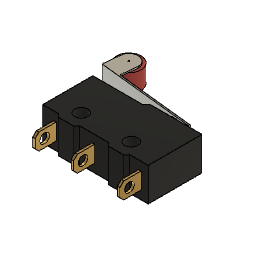
NO-NC Bump Switch (Autodesk Fusion 360 design; units mm, degrees)
Autodesk Fusion 360 part; units mm, degrees
sketch "Body" plane through (0, 0, 0) normal (0, 0, 1) x (1, 0, 0)
  line L0 (10, -5.1) -> (-10, -5.1)
  line L1 (-10, -5.1) -> (-10, 5.1)
  line L2 (-10, 5.1) -> (10, 5.1)
  line L3 (10, 5.1) -> (10, -5.1)
  line L4 (10, -5.1) -> (-10, 5.1) construction
  line L5 (-10, -5.1) -> (10, 5.1) construction
  line L6 (8.4, 5.1) -> (8.4, -5.1) construction
  line L7 (-0.4, 5.1) -> (-0.4, -5.1) construction
  line L8 (-7.7, 5.1) -> (-7.7, -5.1) construction
  line L9 (-7.7, -5.1) -> (-7.7, -9.1) construction
  line L10 (-0.4, -5.1) -> (-0.4, -9.1) construction
  line L11 (8.4, -5.1) -> (8.4, -9.1) construction
  line L12 (-10, -5.1) -> (10, -5.1) construction
  line L13 (10, -5.1) -> (10, -5.71) construction
  line L14 (10, -5.71) -> (-10, -5.71) construction
  line L15 (-10, -5.71) -> (-10, -5.1) construction
  line L16 (10, -2.81) -> (-10, -2.81) construction
  line L17 (-10, -2.81) -> (4.5, -2.81) construction
  circle A0 centre (4.5, -2.81) radius 1.25
  line L18 (4.5, -2.81) -> (-5, -2.81) construction
  circle A1 centre (-5, -2.81) radius 1.25
  line L19 (-5, -2.81) -> (-5, -5.71) construction
  line L20 (4.5, -2.81) -> (4.5, -5.71) construction
  line L21 (3, -5.71) -> (6, -5.71)
  line L22 (4.5, -5.1) -> (4.5, -5.71) construction
  line L23 (-5, -5.1) -> (-5, -5.71) construction
  line L24 (2.5, -5.1) -> (6.5, -5.1)
  line L25 (2.5, -5.1) -> (3, -5.71)
  line L26 (6, -5.71) -> (6.5, -5.1)
  line L27 (-6.5, -5.71) -> (-3.5, -5.71)
  line L28 (-7, -5.1) -> (-3, -5.1)
  line L29 (-7, -5.1) -> (-6.5, -5.71)
  line L30 (-3.5, -5.71) -> (-3, -5.1)
  line L31 (-7.465, -5.1) -> (-7.935, -5.1)
  line L32 (-7.935, -5.1) -> (-7.935, -9.1)
  line L33 (-7.935, -9.1) -> (-7.465, -9.1)
  line L34 (-7.465, -9.1) -> (-7.465, -5.1)
  line L35 (-7.465, -5.1) -> (-7.935, -9.1) construction
  line L36 (-7.935, -5.1) -> (-7.465, -9.1) construction
  line L37 (-0.165, -5.1) -> (-0.635, -5.1)
  line L38 (-0.635, -5.1) -> (-0.635, -9.1)
  line L39 (-0.635, -9.1) -> (-0.165, -9.1)
  line L40 (-0.165, -9.1) -> (-0.165, -5.1)
  line L41 (-0.165, -5.1) -> (-0.635, -9.1) construction
  line L42 (-0.635, -5.1) -> (-0.165, -9.1) construction
  line L43 (8.635, -5.1) -> (8.165, -5.1)
  line L44 (8.165, -5.1) -> (8.165, -9.1)
  line L45 (8.165, -9.1) -> (8.635, -9.1)
  line L46 (8.635, -9.1) -> (8.635, -5.1)
  line L47 (8.635, -5.1) -> (8.165, -9.1) construction
  line L48 (8.165, -5.1) -> (8.635, -9.1) construction
  line L49 (-10, -5.1) -> (-10, 4.38)
  line L50 (-10, 4.38) -> (-0.52, 4.38)
  line L51 (-0.52, 4.38) -> (0.0693, 5.1)
  line L52 (-0.52, 4.38) -> (0.4104, 4.38) construction
  point P0 (4.5, -5.1)
  point P1 (-7.7, -7.1)
  point P2 (-0.4, -7.1)
  point P3 (8.4, -7.1)
  dimension "d1" = 20
  dimension "d2" = 10.2
  dimension "d3" = 1.6
  dimension "d4" = 10.4
  dimension "d5" = 17.7
  dimension "d6" = 4
  dimension "d7" = 4
  dimension "d8" = 4
  dimension "d12" = 0.61
  dimension "d13" = 2.9
  dimension "d14" = 14.5
  dimension "d15" = 2.5
  dimension "d16" = 9.5
  dimension "d17" = 2.5
  dimension "d21" = 3
  dimension "d22" = 4
  dimension "d23" = 3
  dimension "d24" = 4
  dimension "d25" = 0.47
  dimension "d26" = 0.47
  dimension "d27" = 4
  dimension "d28" = 0.47
  dimension "d51" = 9.48
  dimension "d52" = 9.48
  dimension "d53" = 50.7
  constraint horizontal L0
  constraint perpendicular L0 L1
  constraint parallel L0 L2
  constraint parallel L1 L3
  constraint coincident L4 origin
  constraint coincident L5 origin
  constraint perpendicular L0 L9
  constraint perpendicular L0 L10
  constraint perpendicular L0 L11
  constraint horizontal L12
  constraint vertical L13
  constraint horizontal L14
  constraint vertical L15
  constraint coincident L0.start L3.end
  constraint perpendicular L8 L17
  constraint coincident L17.end A0.centre
  constraint parallel L16 L18
  constraint coincident L18.end A1.centre
  constraint coincident L14 L19.end
  constraint perpendicular L14 L19
  constraint coincident L14 L20.end
  constraint perpendicular L14 L20
  constraint coincident L20 P0
  constraint coincident L12 P0
  constraint horizontal L21
  constraint coincident P0 L22.start
  constraint coincident L19 L23.start
  constraint coincident L12 L23.start
  constraint horizontal L24
  constraint midpoint L20.end L21
  constraint midpoint P0 L24
  constraint horizontal L27
  constraint horizontal L28
  constraint midpoint L19.end L27
  constraint midpoint L23.start L28
  constraint horizontal L31
  constraint perpendicular L31 L32
  constraint parallel L31 L33
  constraint parallel L32 L34
  constraint coincident L35 P1
  constraint coincident L36 P1
  constraint midpoint L9 P1
  constraint horizontal L37
  constraint perpendicular L37 L38
  constraint parallel L37 L39
  constraint parallel L38 L40
  constraint coincident L41 P2
  constraint coincident L42 P2
  constraint midpoint L10 P2
  constraint horizontal L43
  constraint perpendicular L43 L44
  constraint parallel L43 L45
  constraint parallel L44 L46
  constraint coincident L47 P3
  constraint coincident L48 P3
  constraint midpoint L11 P3
  constraint perpendicular L16 L49
  constraint perpendicular L8 L50
  constraint horizontal L52
  constraint coincident L2 L51.end
  measures "d1" distance of L1.end L2.end
  measures "d2" distance of L0.end L1.end
  measures "d6" distance of L8.end L9.end
  measures "d7" distance of L7.end L10.end
  measures "d8" distance of L6.end L11.end
  measures "d12" distance of L0.end L14.end
  measures "d14" distance of L16.end L17.end
  measures "d15" diameter of A0
  measures "d16" distance of L17.end L18.end
  measures "d17" diameter of A1
  measures "d21" distance of L21.start L21.end
  measures "d22" distance of L24.start L24.end
  measures "d23" distance of L27.start L27.end
  measures "d24" distance of L28.start L28.end
  measures "d25" distance of L32.end L33.end
  measures "d26" distance of L38.end L39.end
  measures "d27" distance of L37.end L38.end
  measures "d28" distance of L44.end L45.end
  measures "d51" distance of L0.end L49.end
  measures "d52" distance of L49.end L50.end
  measures "d53" angle of L51 L52
sketch "Stem" plane through (0, 0, 0) normal (0, 0, 1) x (1, 0, 0)
  line L0 (2.8, 6.7) -> (3.4, 6.7)
  line L1 (4, 6.1) -> (4, 5.1)
  line L2 (4, 5.1) -> (2.2, 5.1)
  line L3 (2.2, 5.1) -> (2.2, 6.1)
  line L4 (10, 5.1) -> (10, -5.1) construction
  line L5 (10, 5.1) -> (3.1, 5.1) construction
  arc A0 (2.8, 6.7) -> (2.2, 6.1) centre (2.8, 6.1) ccw
  arc A1 (4, 6.1) -> (3.4, 6.7) centre (3.4, 6.1) ccw
  line L6 (10, 5.1) -> (6.4, 5.1) construction
  line L7 (6.4, 5.1) -> (6.4, 4.1) construction
  circle A2 centre (6.4, 4.1) radius 0.125
  line L8 (6.54, 6.2921) -> (6.54, 4.1)
  line L9 (6.54, 4.1) -> (6.26, 4.1)
  line L10 (6.26, 4.1) -> (6.26, 6.2201)
  line L11 (-12.2362, 8.3619) -> (6.0811, 6.419)
  line L12 (-12.2362, 8.3619) -> (-12.2067, 8.6404)
  line L13 (-12.2067, 8.6404) -> (6.1822, 6.6898)
  line L14 (-10, 5.1) -> (10, 5.1)
  line L15 (-12.2362, 8.3619) -> (-11.8671, 11.8424)
  line L16 (-12.2362, 8.3619) -> (-8.7558, 7.9928)
  line L17 (-8.7558, 7.9928) -> (-8.3866, 11.4732)
  line L18 (-10.496, 8.1773) -> (-9.9686, 13.1494) construction
  arc A3 (-8.3866, 11.4732) -> (-11.8671, 11.8424) centre (-10.1554, 11.3885) ccw
  circle A4 centre (-10.1554, 11.3885) radius 0.125
  circle A5 centre (-10.1554, 11.3885) radius 2.31
  arc A6 (6.26, 6.2201) -> (6.0811, 6.419) centre (6.06, 6.2201) ccw
  arc A7 (6.54, 6.2921) -> (6.1822, 6.6898) centre (6.14, 6.2921) ccw
  point P0 (2.2, 6.7)
  point P1 (4, 6.7)
  point P2 (6.26, 6.4)
  point P3 (6.26, 6.4)
  dimension "d29" = 1.8
  dimension "d30" = 1.6
  dimension "d31" = 6.9
  dimension "d32" = 0.6
  dimension "d33" = 3.6
  dimension "d34" = 1
  dimension "d35" = 0.25
  dimension "d39" = 2.3
  dimension "d40" = 18.6
  dimension "d41" = 0.28
  dimension "d42" = 0.28
  dimension "d43" = 3.5
  dimension "d44" = 3.5
  dimension "d45" = 3.5
  dimension "d46" = 5
  dimension "d47" = 0.25
  dimension "d48" = 4.62
  dimension "d49" = 0.2
  dimension "d50" = 0.4
  constraint horizontal L0
  constraint vertical L1
  constraint horizontal L2
  constraint vertical L3
  constraint coincident L4.start L5.start
  constraint perpendicular L4 L5
  constraint midpoint L2 L5.end
  constraint coincident P0 L0
  constraint coincident P0 L3
  constraint tangent L0 A0
  constraint tangent L3 A0
  constraint coincident P1 L0
  constraint coincident P1 L1
  constraint tangent L0 A1
  constraint tangent L1 A1
  constraint equal A0 A1
  constraint perpendicular L4 L6
  constraint perpendicular L6 L7
  constraint coincident L7.end A2.centre
  constraint horizontal L9
  constraint midpoint L7.end L9
  constraint coincident P3 P2
  constraint tangent A1 L11
  constraint perpendicular L11 L12
  constraint perpendicular L12 L13
  constraint perpendicular L8 L14
  constraint perpendicular L10 L14
  constraint perpendicular L13 L15
  constraint coincident L11 L16.end
  constraint perpendicular L13 L17
  constraint midpoint L16 L18.start
  constraint perpendicular L13 L18
  constraint coincident L18.end A3
  constraint concentric A3 A4
  constraint concentric A3 A5
  constraint coincident P3 L11
  constraint coincident P3 L10
  constraint tangent L11 A6
  constraint tangent L10 A6
  constraint tangent L13 A7
  constraint tangent L8 A7
  measures "d29" distance of P0 P1
  measures "d30" distance of P0 L2.end
  measures "d31" distance of L4.start L5.end
  measures "d32" radius of A0
  measures "d33" distance of L4.start L6.end
  measures "d34" distance of L6.end L7.end
  measures "d35" diameter of A2
  measures "d39" distance of P3 L9.end
  measures "d40" distance of L11.start P3
  measures "d41" distance of L11.start L12.end
  measures "d42" distance of L8.end L9.end
  measures "d43" distance of L11.start L15.end
  measures "d44" distance of L11.start L16.end
  measures "d45" distance of L16.end L17.end
  measures "d46" distance of L18.start L18.end
  measures "d47" diameter of A4
  measures "d48" diameter of A5
  measures "d49" radius of A6
  measures "d50" radius of A7
extrude "Extrude1" add sketch "Body" against normal blind 6.34 contours L0 L1 L2 L3 L24 L28 L31 L37 L43 L49 L50 L51 | L0 L21 L24 L25 L26 | L0 L27 L28 L29 L30 makes body 1
extrude "Extrude2" add sketch "Body" against normal blind 6.34 separate body contours L0 L43 L44 L45 L46 | L0 L37 L38 L39 L40 | L0 L31 L32 L33 L34 makes body 2 at (-7.465, -7.7667, -2.1133) makes body 3 at (-0.165, -7.7667, -2.1133) makes body 4 at (8.635, -7.7667, -2.1133)
extrude "Extrude3" add sketch "Stem" against normal blind 6.34 separate body contours L0 L1 L2 L3 A0 A1 L14 makes body 5
extrude "Extrude4" add sketch "Stem" against normal blind 6.34 separate body contours L8 L10 L11 L13 L14 L17 A6 A7 | L11 L12 L13 L15 L16 L17 | L13 L15 L17 A5 | A2 L8 L9 L10 L14 | L15 L17 A3 A5 | A2 L9 picked at (-11.3966, 11.0834) picked at (6.4305, 4.1408) makes body 6
extrude "Extrude5" add sketch "Stem" against normal blind 6.34 separate body contours L15 L17 A3 A5 | L15 L17 A3 A5 makes body 7
sketch "Profile - Contact / Button" plane through (0, 0, 0) normal (1, 0, 0) x (0, 1, 0)
  line L0 (-5.1, 0) -> (-9.1, 0) construction
  line L1 (-9.1, 0) -> (-9.1, -6.34) construction
  line L2 (-9.1, -6.34) -> (-5.1, -6.34) construction
  line L3 (-5.1, -6.34) -> (-5.1, 0) construction
  line L4 (-9.1, -3.17) -> (-5.1, -3.17) construction
  line L5 (-5.1, -4.73) -> (-9.1, -4.73) construction
  line L6 (-9.1, -4.73) -> (-9.1, -1.61) construction
  line L7 (-9.1, -1.61) -> (-5.1, -1.61) construction
  line L8 (-5.1, -1.61) -> (-5.1, -4.73) construction
  line L9 (-5.1, -4.73) -> (-9.1, -1.61) construction
  line L10 (-9.1, -4.73) -> (-5.1, -1.61) construction
  line L11 (-9.1, -3.17) -> (-7.3, -3.17) construction
  circle A0 centre (-7.3, -3.17) radius 0.9
  line L12 (-8.38, -4.73) -> (-8.38, -1.61) construction
  line L13 (-9.1, -2.33) -> (-5.1, -2.33) construction
  line L14 (-5.1, -4.01) -> (-9.1, -4.01) construction
  line L15 (-9.1, -4.01) -> (-8.38, -4.73)
  line L16 (-9.1, -2.33) -> (-8.38, -1.61)
  line L17 (-8.38, -1.61) -> (-5.1, -1.61)
  line L18 (-5.1, -1.61) -> (-5.1, -4.73)
  line L19 (-5.1, -4.73) -> (-8.38, -4.73)
  line L20 (-9.1, -4.01) -> (-9.1, -2.33)
  line L21 (6.7, 0) -> (6.7, -6.34) construction
  line L22 (6.7, 0) -> (6.1, 0) construction
  line L23 (6.1, -6.34) -> (6.7, -6.34) construction
  line L24 (5.1, 0) -> (6.1, 0) construction
  line L25 (5.1, -6.34) -> (6.1, -6.34) construction
  line L26 (5.1, 0) -> (5.1, -6.34) construction
  line L27 (5.1, -3.17) -> (6.7, -3.17) construction
  line L28 (6.7, -4.82) -> (5.1, -4.82)
  line L29 (5.1, -4.82) -> (5.1, -1.52)
  line L30 (5.1, -1.52) -> (6.7, -1.52)
  line L31 (6.7, -1.52) -> (6.7, -4.82)
  line L32 (6.7, -4.82) -> (5.1, -1.52) construction
  line L33 (5.1, -4.82) -> (6.7, -1.52) construction
  point P0 (-7.1, -3.17)
  point P1 (5.9, -3.17)
  dimension "d64" = 3.12
  dimension "d65" = 1.8
  dimension "d66" = 1.8
  dimension "d67" = 0.72
  dimension "d68" = 0.72
  dimension "d69" = 0.72
  dimension "d74" = 3.3
  constraint midpoint L1 L4.start
  constraint midpoint L3 L4.end
  constraint horizontal L5
  constraint perpendicular L5 L6
  constraint parallel L5 L7
  constraint parallel L6 L8
  constraint coincident L9 P0
  constraint coincident L10 P0
  constraint midpoint L4 P0
  constraint coincident L0.start L8
  constraint perpendicular L6 L11
  constraint coincident L11.end A0.centre
  constraint perpendicular L15 L16
  constraint perpendicular L8 L17
  constraint perpendicular L12 L19
  constraint perpendicular L13 L20
  constraint midpoint L26 L27.start
  constraint midpoint L21 L27.end
  constraint horizontal L28
  constraint perpendicular L28 L29
  constraint parallel L28 L30
  constraint parallel L29 L31
  constraint coincident L32 P1
  constraint coincident L33 P1
  constraint midpoint L27 P1
  measures "d64" distance of L5.end L6.end
  measures "d65" distance of L4.start L11.end
  measures "d66" diameter of A0
  measures "d74" distance of L28.end L29.end
extrude "Extrude6" cut sketch "Profile - Contact / Button" against normal blind 10 contours L15 L16 L17 L18 L19 L20 keep common part bodies 2 3
extrude "Extrude7" cut sketch "Profile - Contact / Button" along normal blind 11 contours L15 L16 L17 L18 L19 L20 keep common part bodies 4
extrude "Extrude9" cut sketch "Profile - Contact / Button" along normal blind 6.9 contours L28 L29 L30 L31 keep common part bodies 5
ref_plane "WorkPlane1" through (-0.4282, 15.4359, -3.17) normal (0.10548, 0.994421, 0) x (0.994421, -0.10548, 0)
sketch "Profile - Stem" plane through (-0.4282, 15.4359, -3.17) normal (0.10548, 0.994421, 0) x (0.994421, -0.10548, 0)
  line L0 (-10.996, -3.17) -> (-10.996, 3.17) construction
  line L1 (-10.996, -3.17) -> (7.4241, -3.17) construction
  line L2 (7.4241, 3.17) -> (-10.996, 3.17) construction
  line L3 (7.6229, -3.17) -> (7.4241, -3.17) construction
  line L4 (7.6229, 3.17) -> (7.4241, 3.17) construction
  line L5 (7.8466, -3.17) -> (7.6229, -3.17) construction
  line L6 (7.8466, 3.17) -> (7.6229, 3.17) construction
  line L7 (8.125, -3.17) -> (7.8466, -3.17) construction
  line L8 (8.125, 3.17) -> (7.8466, 3.17) construction
  line L9 (8.125, -3.17) -> (8.125, 3.17) construction
  line L10 (8.125, 0) -> (-10.996, 0) construction
  line L11 (-10.996, 2) -> (8.125, 2)
  line L12 (8.125, 2) -> (8.125, -2)
  line L13 (8.125, -2) -> (-10.996, -2)
  line L14 (-10.996, -2) -> (-10.996, 2)
  line L15 (-10.996, 2) -> (8.125, -2) construction
  line L16 (8.125, 2) -> (-10.996, -2) construction
  line L17 (8.125, -1.72) -> (-10.996, -1.72)
  line L18 (-10.996, 1.72) -> (8.125, 1.72)
  point P0 (-1.4355, 0)
  dimension "d80" = 4
  dimension "d83" = 0.28
  dimension "d84" = 0.28
  constraint midpoint L9 L10.start
  constraint midpoint L0 L10.end
  constraint horizontal L11
  constraint perpendicular L11 L12
  constraint parallel L11 L13
  constraint parallel L12 L14
  constraint coincident L15 P0
  constraint coincident L16 P0
  constraint midpoint L10 P0
  measures "d80" distance of L11.end L12.end
extrude "Extrude10" cut sketch "Profile - Stem" against normal blind 25 keep common part bodies 6
extrude "Extrude12" cut sketch "Profile - Stem" against normal blind 8 contours L12 L14 L17 L18 bodies 6
sketch "Profile - Wheel" plane through (-0.4282, 15.4359, -3.17) normal (0.10548, 0.994421, 0) x (0.994421, -0.10548, 0)
  line L0 (-11.5431, 3.17) -> (-11.556, 3.17)
  line L1 (-6.936, 3.17) -> (-11.5431, 3.17)
  line L2 (-11.5431, -3.17) -> (-6.936, -3.17)
  line L3 (-11.556, -3.17) -> (-11.5431, -3.17)
  line L4 (-6.936, -3.17) -> (-6.936, 3.17)
  line L5 (-11.556, -3.17) -> (-11.556, 3.17)
  line L6 (-10.996, -2) -> (-10.996, 2) construction
  line L7 (-10.996, -2) -> (7.4241, -2) construction
  line L8 (7.4241, -2) -> (7.6229, -2) construction
  line L9 (7.6229, -2) -> (7.8466, -2) construction
  line L10 (7.8466, -2) -> (8.125, -2) construction
  line L11 (7.4241, 2) -> (-10.996, 2) construction
  line L12 (8.125, 2) -> (7.8466, 2) construction
  line L13 (7.8466, 2) -> (7.6229, 2) construction
  line L14 (7.6229, 2) -> (7.4241, 2) construction
  line L15 (8.125, -2) -> (8.125, 2) construction
  line L16 (8.125, -2) -> (-11.556, -2)
  line L17 (8.125, 2) -> (-11.556, 2)
  line L18 (8.125, -1.71) -> (-11.556, -1.71)
  line L19 (8.125, 1.71) -> (-11.556, 1.71)
  dimension "d89" = 0.29
  dimension "d90" = -0.29
  constraint coincident L10.end L15.start
  constraint coincident L5 L16.end
  constraint perpendicular L5 L16
  constraint coincident L12.start L15.end
  constraint coincident L5 L17.end
  constraint perpendicular L5 L17
extrude "Extrude13" cut sketch "Profile - Wheel" against normal blind 8 contours L4 L5 L18 L19 keep common part bodies 7
extrude "Extrude11" [suppressed]
extrude "Extrude8" [suppressed]
equation "d4 = 1.6 mm + 8.8 mm"
equation "d5 = 1.6 mm + 8.8 mm + 7.3 mm"
named bodies: "Body", "Contact 3", "Contact 2", "Contact 1", "Button", "Stem", "Wheel"
